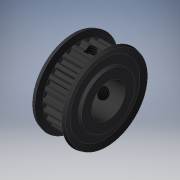
# Autodesk Inventor part: HTPA23S3M060-A-P10_b
Saved by Autodesk Inventor 2019 (Build 230136000, 136)
## iProperties
Created: 2022-11-04
Part Number: HTPA23S3M060-A-P10_b
Material: Generic
Catalog Web Link: www.cadenas.de
Description: HTPA__S3M060, HTPA__S3M100, HTPA__S3M150, HTPB__S3M060, HTPB__S3M100, HTPB__S3M150, HTPK__S3M060, HTPK__S3M100, HTPK__S3M150, HTPN__S3M060, HTPN__S3M100, HTPN__S3M150, HTPT__S3M060, HTPT__S3M100, HTPT__S3M150, HTPM__S3M060, HTPM__S3M100, HTPM__S3M150, HTPP__S3M060, HTPP__S3M100, HTPP__S3M150, HTPS__S3M060, HTPS__S3M100, KHTPA__S3M060, KHTPA__S3M100, KHTPA__S3M150, KHTPK__S3M060, KHTPK__S3M100, KHTPK__S3M150_body-High Torque Timing Pulleys S3M Type
Vendor: MISUMI
Document SubType Name: Modeling
Designer: psAdmin
Manufacturer: MISUMI
Mass: 2.63016 g
Surface Area: 24.7129 cm^2
Volume: 2.63016 cm^3
Density: 1 g/cm^3
Appearance: PSOLRGB-175-175-175
Category: PARTsolutions
Company: MISUMI
Title: HTPA23S3M060-A-P10
Author: Cadenas PARTsolutions
Comments: High Torque Timing Pulleys S3M Type
PSOL_IDENT_0: {$CADENAS_DATA/23d-libs/misumi/metric/51_timing_pulleys/htpk_s3m/htpa_s3m.prj},837 {VTYP=3D},{NB=HTP
PSOL_IDENT_1: A23S3M060-A-P10_b},{LINA=HTPA23S3M060-A-P10},{NN=HTPA__S3M060, HTPA__S3M100, HTPA__S3M150, HTPB__S3M
PSOL_IDENT_2: 060, HTPB__S3M100, HTPB__S3M150, HTPK__S3M060, HTPK__S3M100, HTPK__S3M150, HTPN__S3M060, HTPN__S3M10
PSOL_IDENT_3: 0, HTPN__S3M150, HTPT__S3M060, HTPT__S3M100, HTPT__S3M150, HTPM__S3M060, HTPM__S3M100, HTPM__S3M150,
PSOL_IDENT_4: HTPP__S3M060, HTPP__S3M100, HTPP__S3M150, HTPS__S3M060, HTPS__S3M100, KHTPA__S3M060, KHTPA__S3M100,
PSOL_IDENT_5: KHTPA__S3M150, KHTPK__S3M060, KHTPK__S3M100, KHTPK__S3M150_body},{DATE=28.10.2022 00:10:57},{GEOMDA
PSOL_IDENT_6: TE=11.11.2021 09:52:43},{VERSION=},{LINEID=330},{WBVAR=MATP,ST,TNW,PS,SBS,DD,Z,J,Q,R,S,T,ALT1,ALT2,M
PSOL_IDENT_7: ,QSC,QFC,QTC,ALT3,K,KSC,KFC,KTC,ALT4,ZM,ZSC,ZFC,ZTC,ALT5,ALT6,ALT7,FC,ALT8,SRG,ALT9,BTC,TL,ALT10,TPC
PSOL_IDENT_8: ,ALT11,BC,ALT12,SLH,ALT13,BN},{WBNUMERIC=DD,Z,J,Q,R,S,T,QSC,QFC,QTC,K,KSC,KFC,KTC,ZSC,ZFC,ZTC,FC,SRG
PSOL_IDENT_9: ,BTC,TL,BC,SLH,BN}  {NB=HTPA23S3M060-A-P10_b},{LINA=HTPA23S3M060-A-P10},{KT=DUMMY},{PN=HTPA23S3M060-
PSOL_IDENT_10: A-P10},{TYPE=HTPA},{MATP=A2017},{MATPALG='A2017','Aluminum Alloy 2000 series','S45C','1045 Carbon St
PSOL_IDENT_11: eel Equivalent','SUS304','304 Stainless Steel','A6000','6000 Series Aluminum Alloy'},{ST=CA},{STALG=
PSOL_IDENT_12: 'CA','Clear Anodize','BA','Black Anodize','HAT','Hard Clear Anodize','ENP','Electroless Nickel Plat
PSOL_IDENT_13: ing' },{NT=23},{TNW=S3M060},{TNWALG= 'S3M060','S3M100','S3M150'    },{BW=6},{PS=A},{PSALG='A','B'},{
PSOL_IDENT_14: SBS=P},{SBSALG= 'H','Round Hole','P','Round Hole + Tap','V','Stepped Hole', 'Y','Both Ends Stepped H
PSOL_IDENT_15: ole','WB', 'Double Stepped Hole' },{SHSA= 'H','Round Hole','P','Round Hole + Tap','V','Stepped Hole'
PSOL_IDENT_16: , 'Y','Both Ends Stepped Hole','WB', 'Double Stepped Hole' },{SHSB= 'H','Round Hole','P','Round Hole
PSOL_IDENT_17: + Tap','V','Stepped Hole','F','Stepped Hole (Counterbore holes on the boss side)'},{SHSK='H','Round
PSOL_IDENT_18: Hole','P','Round Hole + Tap'},{SBSPN=-P10},{DD=10.00},{DDALG=[4:4/1],4.5,[5:6/1],6.35,[7:10/1]},{DD
PSOL_IDENT_19: HA=[4:4/1],4.5,[5:6/1],6.35,[7:12/1]},{DDHBK=0},{DDPA=[4:4/1],4.5,[5:6/1],6.35,[7:10/1]},{DDPBK=0},{
PSOL_IDENT_20: DDNA=[8:8/1],[10:11/1]},{DDNBK=0},{DDNK=0},{DDCA=[10:10/1]},{DDCBK=0},{DDVA=[4:4/1],4.5,[5:6/1],6.35
PSOL_IDENT_21: ,[7:10/1]},{DDVF=[4:4/1],4.5,[5:6/1],6.35,[7:8/1]},{DDY=[4:10/1]},{DDWB=[4:8/1]},{Z=0},{ZALG=[0]},{Z
PSOL_IDENT_22: QRMIN=12},{ZAMAX=12},{ZBMAX=10},{DDZ=10},{J=0.0},{JALG=[0]},{JMAX=9},{JMIN=2},{JPN=},{QRMAX=12},{QRM
PSOL_IDENT_23: IN=12},{WBRMAX=-2.00},{WBQMIN=14},{Q=0},{QALG=[0]},{QPN=},{R=0},{RALG=[0]},{S=0.0},{SALG=[0]},{SPN=}
PSOL_IDENT_24: ,{SMAX=5},{T=0.0},{TALG=[0]},{TPN=},{TMAX=8},{A=7},{W=11},{L=0},{PD=21.96},{OD=21.20},{D=0},{DALG=25
PSOL_IDENT_25: },{DE=16},{F=25},{E=16},{BBK=0.000},{TTK=0.0},{TT=1},{ANG=125.217391},{WL=11},{ALT1=},{ALT1ALG= '','
PSOL_IDENT_26: w/o KC90 (Set Screw Angle)','KC90','with KC90 (Set Screw Angle)' },{ALT1PN=},{ALT2=},{ALT2ALG= '','N
PSOL_IDENT_27: ot applicable' },{M=N/A},{MALG= 'N/A' },{MFTALG= 'N/A' },{MSALG= 'N/A' },{M3D=0.000},{KDML=0},{ML=0}
PSOL_IDENT_28: ,{MUL=0},{PITCH=0},{QSC=0.0},{QSCALG=0},{QFC=0.0},{QFCALG=0},{QTC=0.0},{QTCALG=0},{QPCDMIN=0},{QPCDM
PSOL_IDENT_29: INALG=0},{QPCDMAX=12},{ALT2PN=},{ALT3=},{ALT3ALG= '','Not applicable' },{K=0.0},{KALG=0},{KMIN=4},{K
PSOL_IDENT_30: FTMAX=0.0},{KSMAX=0.0},{KSC=0.0},{KSCALG=0},{KFC=0.0},{KFCALG=0},{KTC=0.0},{KTCALG=0},{KPCDMIN=14},{
PSOL_IDENT_31: KPCDMINALG=14},{KPCDMAX=12},{KSCMIN=14.0},{KSCMINALG=14},{ALT3PN=},{ALT4=},{ALT4ALG= '','Not applica
PSOL_IDENT_32: ble' },{ALT4MIN=20.5},{ALT4MAX=5.5},{ZM=N/A},{ZMALG= 'N/A' },{ZMSALG= 'N/A' },{ZMFTALG= 'N/A' },{ZMD
PSOL_IDENT_33: D1=0.0},{ZMDD2=0.0},{ZMHH=0.0},{ZSC=0.0},{ZSCALG=[0]},{ZFC=0.0},{ZFCALG=[0]},{ZTC=0.0},{ZTCALG=[0]},
PSOL_IDENT_34: {ZPCDMIN=0},{ZPCDMINALG=0},{ZPCDMAX=12},{ALT4PN=},{ALT5=},{ALT5ALG= '','Flange Attached','NFC','with
PSOL_IDENT_35: NFC (Flange not Attached)' },{ALT5PN=},{ALT6=},{ALT6ALG= '','w/o Flange Attached on One Side Only','
PSOL_IDENT_36: RFC','with RFC (Flange Attached on The Boss Side Only)','LFC','with LFC (Flange Attached on The Oppo
PSOL_IDENT_37: site Side Only)' },{ALT6PN=},{ALT7=},{ALT7ALG= '','w/o FC (Flange Cut)','FC','with FC (Flange Cut)'
PSOL_IDENT_38: },{FC=0.0},{FCALG=0},{FCMIN=22.5},{FCMAX=23.0},{ALT7PN=},{ALT8=},{ALT8ALG= '','Not applicable' },{AL
PSOL_IDENT_39: T8ALGALG=12},{ALT8DD2=0},{ALT8MM=0},{ALT8NN=0},{QC=0},{KC=0},{ZC=0},{SRG=0.0},{SRGALG=[0]},{SRGMAX1=
PSOL_IDENT_40: 0},{SRGMAX=0},{DD2=0.0},{MM=0.00},{NN=0.00},{ALT8PN=},{ALT9ALG= '','w/o BTC (Taper for Bearing Holde
PSOL_IDENT_41: r)','BTC','with BTC (Taper for Bearing Holder)' },{ALT9=},{BTC9=11},{TL9=1},{BTC=0},{BTCALG=[0]},{TL=
PSOL_IDENT_42: 0.0},{TLALG=0},{TLMIN=1.0},{TLMAX=-11.5},{BTCL=0},{BTCD=0},{BTCDALG=16.000},{ALT9PN=},{WLBCTL=11},{A
PSOL_IDENT_43: LT10=},{ALT10ALG= '','w/o TPC (Tapped Hole Dimension)','TPC','with TPC (Tapped Hole Dimension)' },{T
PSOL_IDENT_44: PC=N/A},{TPCALG= 'N/A' },{TPCM=4},{ALT10PN=},{ALT11=},{ALT11ALG= '','Not applicable' },{BC=0.0},{BCA
PSOL_IDENT_45: LG=0},{BCMIN=7},{BCMAX=-11.5},{BCPLANE=5.5},{M1WBC=5.5},{ALT11PN=},{ALT12=},{ALT12ALG= '','w/o SLH (
PSOL_IDENT_46: Set Screw Length)','SLH','with SLH (Set Screw Length)' },{SLH=0},{SLHALG=[0]},{ALT12PN=},{AC=M4x3},{
PSOL_IDENT_47: M1=4},{M1L=3},{TAP=0.000},{KYY=5},{KTT=5.6},{PLANE=11},{CD=0},{ALT13=},{ALT13ALG= '', 'Not applicabl
PSOL_IDENT_48: e' },{BN=0.0},{BNALG=0},{BNMIN=-10.5},{BNMAX=-1.0},{ALT13PN=}
NB: HTPA23S3M060-A-P10_b
NN: 0
NT: 23
NBSYN: $PN._b
LINA: HTPA23S3M060-A-P10
CATALOG: Misumi
PN: HTPA23S3M060-A-P10
MATP: Aluminum Alloy 2000 series
ST: Clear Anodize
TNW: S3M060
BW: 6
PS: A
SBS: Round Hole + Tap
DD: 10
Z: 0
J: 0
Q: 0
R: 0
S: 0
T: 0
A: 7
W: 11
L: 0
PD: 21.96
OD: 21.2
D: 0
F: 25
E: 16
TT: 1
ALT1: w/o KC90 (Set Screw Angle)
ALT2: Not applicable
M: N/A
QSC: 0
QFC: 0
QTC: 0
ALT3: Not applicable
K: 0
KSC: 0
KFC: 0
KTC: 0
ALT4: Not applicable
ZM: N/A
ZMDD1: 0
ZMDD2: 0
ZMHH: 0
ZSC: 0
ZFC: 0
ZTC: 0
ALT5: Flange Attached
ALT6: w/o Flange Attached on One Side Only
ALT7: w/o FC (Flange Cut)
FC: 0
ALT8: Not applicable
SRG: 0
DD2: 0
MM: 0
ALT9: w/o BTC (Taper for Bearing Holder)
BTC: 0
TL: 0
BTCL: 0
BTCD: 0
ALT10: w/o TPC (Tapped Hole Dimension)
TPC: N/A
ALT11: Not applicable
BC: 0
ALT12: w/o SLH (Set Screw Length)
SLH: 0
AC: M4x3
ALT13: Not applicable
BN: 0
SUPPLIER: MISUMI
ARTICLENO: HTPA23S3M060-A-P10_b
BOMINFO: HTPA23S3M060-A-P10
CREATOR: CADENAS GmbH
Autodesk Inventor part; units mm, degrees
ref_plane "YZ Plane" through (0, 0, 0) normal (1, 0, 0) x (0, 1, 0)
ref_plane "XZ Plane" through (0, 0, 0) normal (0, 1, 0) x (-1, 0, 0)
ref_plane "XY Plane" through (0, 0, 0) normal (0, 0, 1) x (1, 0, 0)
sketch "_____1" plane through (0, 0, 0) normal (0, 0, 1) x (1, 0, 0)
  line L0 (11, 0) -> (0, 0)
  line L1 (0, 0) -> (0, 8)
  line L2 (0, 8) -> (1, 8)
  line L3 (1, 8) -> (1, 10.4683)
  line L4 (1, 10.4683) -> (0.525, 12.2412)
  line L5 (0.525, 12.2412) -> (1.4909, 12.5)
  line L6 (1.4909, 12.5) -> (2, 10.6)
  line L7 (2, 10.6) -> (9, 10.6)
  line L8 (9, 10.6) -> (9.5091, 12.5)
  line L9 (9.5091, 12.5) -> (10.475, 12.2412)
  line L10 (10.475, 12.2412) -> (10, 10.4683)
  line L11 (10, 10.4683) -> (10, 8)
  line L12 (10, 8) -> (11, 8)
  line L13 (11, 8) -> (11, 0)
  line L14 (11, 0) -> (0, 0)
  constraints: 30 end point
revolve "Revolution1" add sketch "_____1" angle 360 about axis through (11, 0, 0) along (1, 0, 0)
sketch "Sketch2" plane through (11, 0, 0) normal (1, 0, 0) x (0, 0, -1)
  point P0 (0, 0)
hole "Hole1" at (11, 0, 0) direction (-1, 0, 0) diameter 10 depth 11
sketch "_____6" plane through (2, 0, 0) normal (1, 0, 0) x (0, 0, -1)
  circle A0 centre (0, 0) radius 15.6
  arc A1 (-10.5889, 0.4842) -> (-10.3757, 0.1995) centre (-10.3092, 0.4715) ccw
  arc A2 (-9.534, -0.2416) -> (-10.3757, 0.1995) centre (-10.8446, -1.7191) ccw
  arc A3 (-9.4836, -0.3483) -> (-9.534, -0.2416) centre (-9.6335, -0.3538) ccw
  arc A4 (-9.4836, -0.3483) -> (-9.4427, -0.9463) centre (0, 0) ccw
  arc A5 (-9.4781, -1.0588) -> (-9.4427, -0.9463) centre (-9.592, -0.9612) ccw
  arc A6 (-10.2519, -1.6104) -> (-9.4781, -1.0588) centre (-10.9777, 0.2264) ccw
  arc A7 (-10.2519, -1.6104) -> (-10.4244, -1.9216) centre (-10.149, -1.8708) ccw
  arc A8 (-10.4244, -1.9216) -> (-10.3269, -2.3906) centre (0, 0) ccw
  arc A9 (-10.3269, -2.3906) -> (-10.0448, -2.6073) centre (-10.0541, -2.3274) ccw
  arc A10 (-9.1152, -2.8049) -> (-10.0448, -2.6073) centre (-9.9786, -4.5812) ccw
  arc A11 (-9.038, -2.894) -> (-9.1152, -2.8049) centre (-9.1808, -2.9398) ccw
  arc A12 (-9.038, -2.894) -> (-8.8372, -3.4588) centre (0, 0) ccw
  arc A13 (-8.8409, -3.5767) -> (-8.8372, -3.4588) centre (-8.9769, -3.5135) ccw
  arc A14 (-9.4372, -4.3166) -> (-8.8409, -3.5767) centre (-10.6317, -2.7437) ccw
  arc A15 (-9.4372, -4.3166) -> (-9.5194, -4.6628) centre (-9.2679, -4.5396) ccw
  arc A16 (-9.5194, -4.6628) -> (-9.299, -5.0881) centre (0, 0) ccw
  arc A17 (-9.299, -5.0881) -> (-8.9688, -5.2206) centre (-9.0534, -4.9537) ccw
  arc A18 (-8.0205, -5.1601) -> (-8.9688, -5.2206) centre (-8.3726, -7.1035) ccw
  arc A19 (-7.922, -5.2251) -> (-8.0205, -5.1601) centre (-8.0472, -5.3077) ccw
  arc A20 (-7.922, -5.2251) -> (-7.5764, -5.7148) centre (0, 0) ccw
  arc A21 (-7.5481, -5.8293) -> (-7.5764, -5.7148) centre (-7.6961, -5.8051) ccw
  arc A22 (-7.9227, -6.7027) -> (-7.5481, -5.8293) centre (-9.4972, -5.5104) ccw
  arc A23 (-7.9227, -6.7027) -> (-7.9084, -7.0582) centre (-7.6995, -6.8717) ccw
  arc A24 (-7.9084, -7.0582) -> (-7.5814, -7.4082) centre (0, 0) ccw
  arc A25 (-7.5814, -7.4082) -> (-7.2277, -7.4468) centre (-7.3812, -7.2126) ccw
  arc A26 (-6.3309, -7.1327) -> (-7.2277, -7.4468) centre (-6.1457, -9.099) ccw
  arc A27 (-6.2185, -7.1687) -> (-6.3309, -7.1327) centre (-6.3168, -7.282) ccw
  arc A28 (-6.2185, -7.1687) -> (-5.7536, -7.547) centre (0, 0) ccw
  arc A29 (-5.6954, -7.6496) -> (-5.7536, -7.547) centre (-5.8445, -7.6662) ccw
  arc A30 (-5.8205, -8.5917) -> (-5.6954, -7.6496) centre (-7.6583, -7.8684) ccw
  arc A31 (-5.8205, -8.5917) -> (-5.7108, -8.9301) centre (-5.56, -8.6942) ccw
  arc A32 (-5.7108, -8.9301) -> (-5.3016, -9.179) centre (0, 0) ccw
  arc A33 (-5.3016, -9.179) -> (-4.9506, -9.1207) centre (-5.1615, -8.9365) ccw
  arc A34 (-4.1717, -8.5762) -> (-4.9506, -9.1207) centre (-3.4629, -10.4196) ccw
  arc A35 (-4.0538, -8.5806) -> (-4.1717, -8.5762) centre (-4.1179, -8.7162) ccw
  arc A36 (-4.0538, -8.5806) -> (-3.5041, -8.8194) centre (0, 0) ccw
  arc A37 (-3.4204, -8.9026) -> (-3.5041, -8.8194) centre (-3.5595, -8.9588) ccw
  arc A38 (-3.2867, -9.8434) -> (-3.4204, -8.9026) centre (-5.2514, -9.6428) ccw
  arc A39 (-3.2867, -9.8434) -> (-3.0897, -10.1397) centre (-3.0081, -9.8719) ccw
  arc A40 (-3.0897, -10.1397) -> (-2.6285, -10.2689) centre (0, 0) ccw
  arc A41 (-2.6285, -10.2689) -> (-2.3063, -10.1181) centre (-2.5591, -9.9977) ccw
  arc A42 (-1.7032, -9.3837) -> (-2.3063, -10.1181) centre (-0.5233, -10.9675) ccw
  arc A43 (-1.5885, -9.3561) -> (-1.7032, -9.3837) centre (-1.6136, -9.504) ccw
  arc A44 (-1.5885, -9.3561) -> (-0.9947, -9.4377) centre (0, 0) ccw
  arc A45 (-0.8917, -9.4952) -> (-0.9947, -9.4377) centre (-1.0104, -9.5869) ccw
  arc A46 (-0.5091, -10.3651) -> (-0.8917, -9.4952) centre (-2.4551, -10.702) ccw
  arc A47 (-0.5091, -10.3651) -> (-0.2395, -10.5973) centre (-0.2332, -10.3174) ccw
  arc A48 (-0.2395, -10.5973) -> (0.2395, -10.5973) centre (0, 0) ccw
  arc A49 (0.2395, -10.5973) -> (0.5091, -10.3651) centre (0.2332, -10.3174) ccw
  arc A50 (0.8917, -9.4952) -> (0.5091, -10.3651) centre (2.4551, -10.702) ccw
  arc A51 (0.9947, -9.4377) -> (0.8917, -9.4952) centre (1.0104, -9.5869) ccw
  arc A52 (0.9947, -9.4377) -> (1.5885, -9.3561) centre (0, 0) ccw
  arc A53 (1.7032, -9.3837) -> (1.5885, -9.3561) centre (1.6136, -9.504) ccw
  arc A54 (2.3063, -10.1181) -> (1.7032, -9.3837) centre (0.5233, -10.9675) ccw
  arc A55 (2.3063, -10.1181) -> (2.6285, -10.2689) centre (2.5591, -9.9977) ccw
  arc A56 (2.6285, -10.2689) -> (3.0897, -10.1397) centre (0, 0) ccw
  arc A57 (3.0897, -10.1397) -> (3.2867, -9.8434) centre (3.0081, -9.8719) ccw
  arc A58 (3.4204, -8.9026) -> (3.2867, -9.8434) centre (5.2514, -9.6428) ccw
  arc A59 (3.5041, -8.8194) -> (3.4204, -8.9026) centre (3.5595, -8.9588) ccw
  arc A60 (3.5041, -8.8194) -> (4.0538, -8.5806) centre (0, 0) ccw
  arc A61 (4.1717, -8.5762) -> (4.0538, -8.5806) centre (4.1179, -8.7162) ccw
  arc A62 (4.9506, -9.1207) -> (4.1717, -8.5762) centre (3.4629, -10.4196) ccw
  arc A63 (4.9506, -9.1207) -> (5.3016, -9.179) centre (5.1615, -8.9365) ccw
  arc A64 (5.3016, -9.179) -> (5.7108, -8.9301) centre (0, 0) ccw
  arc A65 (5.7108, -8.9301) -> (5.8205, -8.5917) centre (5.56, -8.6942) ccw
  arc A66 (5.6954, -7.6496) -> (5.8205, -8.5917) centre (7.6583, -7.8684) ccw
  arc A67 (5.7536, -7.547) -> (5.6954, -7.6496) centre (5.8445, -7.6662) ccw
  arc A68 (5.7536, -7.547) -> (6.2185, -7.1687) centre (0, 0) ccw
  arc A69 (6.3309, -7.1327) -> (6.2185, -7.1687) centre (6.3168, -7.282) ccw
  arc A70 (7.2277, -7.4468) -> (6.3309, -7.1327) centre (6.1457, -9.099) ccw
  arc A71 (7.2277, -7.4468) -> (7.5814, -7.4082) centre (7.3812, -7.2126) ccw
  arc A72 (7.5814, -7.4082) -> (7.9084, -7.0582) centre (0, 0) ccw
  arc A73 (7.9084, -7.0582) -> (7.9227, -6.7027) centre (7.6995, -6.8717) ccw
  arc A74 (7.5481, -5.8293) -> (7.9227, -6.7027) centre (9.4972, -5.5104) ccw
  arc A75 (7.5764, -5.7148) -> (7.5481, -5.8293) centre (7.6961, -5.8051) ccw
  arc A76 (7.5764, -5.7148) -> (7.922, -5.2251) centre (0, 0) ccw
  arc A77 (8.0205, -5.1601) -> (7.922, -5.2251) centre (8.0472, -5.3077) ccw
  arc A78 (8.9688, -5.2206) -> (8.0205, -5.1601) centre (8.3726, -7.1035) ccw
  arc A79 (8.9688, -5.2206) -> (9.299, -5.0881) centre (9.0534, -4.9537) ccw
  arc A80 (9.299, -5.0881) -> (9.5194, -4.6628) centre (0, 0) ccw
  arc A81 (9.5194, -4.6628) -> (9.4372, -4.3166) centre (9.2679, -4.5396) ccw
  arc A82 (8.8409, -3.5767) -> (9.4372, -4.3166) centre (10.6317, -2.7437) ccw
  arc A83 (8.8372, -3.4588) -> (8.8409, -3.5767) centre (8.9769, -3.5135) ccw
  arc A84 (8.8372, -3.4588) -> (9.038, -2.894) centre (0, 0) ccw
  arc A85 (9.1152, -2.8049) -> (9.038, -2.894) centre (9.1808, -2.9398) ccw
  arc A86 (10.0448, -2.6073) -> (9.1152, -2.8049) centre (9.9786, -4.5812) ccw
  arc A87 (10.0448, -2.6073) -> (10.3269, -2.3906) centre (10.0541, -2.3274) ccw
  arc A88 (10.3269, -2.3906) -> (10.4244, -1.9216) centre (0, 0) ccw
  arc A89 (10.4244, -1.9216) -> (10.2519, -1.6104) centre (10.149, -1.8708) ccw
  arc A90 (9.4781, -1.0588) -> (10.2519, -1.6104) centre (10.9777, 0.2264) ccw
  arc A91 (9.4427, -0.9463) -> (9.4781, -1.0588) centre (9.592, -0.9612) ccw
  arc A92 (9.4427, -0.9463) -> (9.4836, -0.3483) centre (0, 0) ccw
  arc A93 (9.534, -0.2416) -> (9.4836, -0.3483) centre (9.6335, -0.3538) ccw
  arc A94 (10.3757, 0.1995) -> (9.534, -0.2416) centre (10.8446, -1.7191) ccw
  arc A95 (10.3757, 0.1995) -> (10.5889, 0.4842) centre (10.3092, 0.4715) ccw
  arc A96 (10.5889, 0.4842) -> (10.5562, 0.9621) centre (0, 0) ccw
  arc A97 (10.5562, 0.9621) -> (10.3062, 1.2152) centre (10.2774, 0.9367) ccw
  arc A98 (9.4123, 1.5376) -> (10.3062, 1.2152) centre (10.5095, 3.1797) ccw
  arc A99 (9.3478, 1.6364) -> (9.4123, 1.5376) centre (9.4956, 1.6623) ccw
  arc A100 (9.3478, 1.6364) -> (9.2259, 2.2232) centre (0, 0) ccw
  arc A101 (9.2456, 2.3396) -> (9.2259, 2.2232) centre (9.3717, 2.2584) ccw
  arc A102 (9.9371, 2.9914) -> (9.2456, 2.3396) centre (10.9062, 1.2705) ccw
  arc A103 (9.9371, 2.9914) -> (10.0656, 3.3232) centre (9.7997, 3.2354) ccw
  arc A104 (10.0656, 3.3232) -> (9.9052, 3.7745) centre (0, 0) ccw
  arc A105 (9.9052, 3.7745) -> (9.5962, 3.9507) centre (9.6436, 3.6748) ccw
  arc A106 (8.6484, 4.02) -> (9.5962, 3.9507) centre (9.2619, 5.8972) ccw
  arc A107 (8.5597, 4.0978) -> (8.6484, 4.02) centre (8.695, 4.1625) ccw
  arc A108 (8.5597, 4.0978) -> (8.284, 4.6299) centre (0, 0) ccw
  arc A109 (8.2715, 4.7473) -> (8.284, 4.6299) centre (8.4149, 4.7031) ccw
  arc A110 (8.7616, 5.5615) -> (8.2715, 4.7473) centre (10.159, 4.1659) ccw
  arc A111 (8.7616, 5.5615) -> (8.7958, 5.9156) centre (8.5634, 5.7593) ccw
  arc A112 (8.7958, 5.9156) -> (8.5196, 6.3069) centre (0, 0) ccw
  arc A113 (8.5196, 6.3069) -> (8.1744, 6.3933) centre (8.2945, 6.1403) ccw
  arc A114 (7.2431, 6.2042) -> (8.1744, 6.3933) centre (7.3274, 8.1774) ccw
  arc A115 (7.1367, 6.2552) -> (7.2431, 6.2042) centre (7.2495, 6.3541) ccw
  arc A116 (7.1367, 6.2552) -> (6.7276, 6.6932) centre (0, 0) ccw
  arc A117 (6.684, 6.8028) -> (6.7276, 6.6932) centre (6.834, 6.799) ccw
  arc A118 (6.9362, 7.7191) -> (6.684, 6.8028) centre (8.6584, 6.7523) ccw
  arc A119 (6.9362, 7.7191) -> (6.8736, 8.0693) centre (6.692, 7.8561) ccw
  arc A120 (6.8736, 8.0693) -> (6.502, 8.3716) centre (0, 0) ccw
  arc A121 (6.502, 8.3716) -> (6.1464, 8.3616) centre (6.3303, 8.1504) ccw
  arc A122 (5.3007, 7.9283) -> (6.1464, 8.3616) centre (4.8494, 9.8511) ccw
  arc A123 (5.1844, 7.9487) -> (5.3007, 7.9283) centre (5.2664, 8.0743) ccw
  arc A124 (5.1844, 7.9487) -> (4.6723, 8.2601) centre (0, 0) ccw
  arc A125 (4.6008, 8.3539) -> (4.6723, 8.2601) centre (4.7462, 8.3907) ccw
  arc A126 (4.5964, 9.3042) -> (4.6008, 8.3539) centre (6.5156, 8.8379) ccw
  arc A127 (4.5964, 9.3042) -> (4.4416, 9.6245) centre (4.3243, 9.3703) ccw
  arc A128 (4.4416, 9.6245) -> (4.0023, 9.8154) centre (0, 0) ccw
  arc A129 (4.0023, 9.8154) -> (3.6626, 9.7098) centre (3.8966, 9.5561) ccw
  arc A130 (2.9651, 9.0644) -> (3.6626, 9.7098) centre (2.0118, 10.7941) ccw
  arc A131 (2.8477, 9.0527) -> (2.9651, 9.0644) centre (2.8927, 9.1958) ccw
  arc A132 (2.8477, 9.0527) -> (2.2705, 9.2144) centre (0, 0) ccw
  arc A133 (2.1763, 9.2854) -> (2.2705, 9.2144) centre (2.3064, 9.36) ccw
  arc A134 (1.9157, 10.1993) -> (2.1763, 9.2854) centre (3.8895, 10.268) ccw
  arc A135 (1.9157, 10.1993) -> (1.6803, 10.466) centre (1.6359, 10.1895) ccw
  arc A136 (1.6803, 10.466) -> (1.2057, 10.5312) centre (0, 0) ccw
  arc A137 (1.2057, 10.5312) -> (0.9071, 10.3379) centre (1.1739, 10.253) ccw
  arc A138 (0.4096, 9.5282) -> (0.9071, 10.3379) centre (-0.975, 10.9366) ccw
  arc A139 (0.2997, 9.4853) -> (0.4096, 9.5282) centre (0.3044, 9.6352) ccw
  arc A140 (0.2997, 9.4853) -> (-0.2997, 9.4853) centre (0, 0) ccw
  arc A141 (-0.4096, 9.5282) -> (-0.2997, 9.4853) centre (-0.3044, 9.6352) ccw
  arc A142 (-0.9071, 10.3379) -> (-0.4096, 9.5282) centre (0.975, 10.9366) ccw
  arc A143 (-0.9071, 10.3379) -> (-1.2057, 10.5312) centre (-1.1739, 10.253) ccw
  arc A144 (-1.2057, 10.5312) -> (-1.6803, 10.466) centre (0, 0) ccw
  arc A145 (-1.6803, 10.466) -> (-1.9157, 10.1993) centre (-1.6359, 10.1895) ccw
  arc A146 (-2.1763, 9.2854) -> (-1.9157, 10.1993) centre (-3.8895, 10.268) ccw
  arc A147 (-2.2705, 9.2144) -> (-2.1763, 9.2854) centre (-2.3064, 9.36) ccw
  arc A148 (-2.2705, 9.2144) -> (-2.8477, 9.0527) centre (0, 0) ccw
  arc A149 (-2.9651, 9.0644) -> (-2.8477, 9.0527) centre (-2.8927, 9.1958) ccw
  arc A150 (-3.6626, 9.7098) -> (-2.9651, 9.0644) centre (-2.0118, 10.7941) ccw
  arc A151 (-3.6626, 9.7098) -> (-4.0023, 9.8154) centre (-3.8966, 9.5561) ccw
  arc A152 (-4.0023, 9.8154) -> (-4.4416, 9.6245) centre (0, 0) ccw
  arc A153 (-4.4416, 9.6245) -> (-4.5964, 9.3042) centre (-4.3243, 9.3703) ccw
  arc A154 (-4.6008, 8.3539) -> (-4.5964, 9.3042) centre (-6.5156, 8.8379) ccw
  arc A155 (-4.6723, 8.2601) -> (-4.6008, 8.3539) centre (-4.7462, 8.3907) ccw
  arc A156 (-4.6723, 8.2601) -> (-5.1844, 7.9487) centre (0, 0) ccw
  arc A157 (-5.3007, 7.9283) -> (-5.1844, 7.9487) centre (-5.2664, 8.0743) ccw
  arc A158 (-6.1464, 8.3616) -> (-5.3007, 7.9283) centre (-4.8494, 9.8511) ccw
  arc A159 (-6.1464, 8.3616) -> (-6.502, 8.3716) centre (-6.3303, 8.1504) ccw
  arc A160 (-6.502, 8.3716) -> (-6.8736, 8.0693) centre (0, 0) ccw
  arc A161 (-6.8736, 8.0693) -> (-6.9362, 7.7191) centre (-6.692, 7.8561) ccw
  arc A162 (-6.684, 6.8028) -> (-6.9362, 7.7191) centre (-8.6584, 6.7523) ccw
  arc A163 (-6.7276, 6.6932) -> (-6.684, 6.8028) centre (-6.834, 6.799) ccw
  arc A164 (-6.7276, 6.6932) -> (-7.1367, 6.2552) centre (0, 0) ccw
  arc A165 (-7.2431, 6.2042) -> (-7.1367, 6.2552) centre (-7.2495, 6.3541) ccw
  arc A166 (-8.1744, 6.3933) -> (-7.2431, 6.2042) centre (-7.3274, 8.1774) ccw
  arc A167 (-8.1744, 6.3933) -> (-8.5196, 6.3069) centre (-8.2945, 6.1403) ccw
  arc A168 (-8.5196, 6.3069) -> (-8.7958, 5.9156) centre (0, 0) ccw
  arc A169 (-8.7958, 5.9156) -> (-8.7616, 5.5615) centre (-8.5634, 5.7593) ccw
  arc A170 (-8.2715, 4.7473) -> (-8.7616, 5.5615) centre (-10.159, 4.1659) ccw
  arc A171 (-8.284, 4.6299) -> (-8.2715, 4.7473) centre (-8.4149, 4.7031) ccw
  arc A172 (-8.284, 4.6299) -> (-8.5597, 4.0978) centre (0, 0) ccw
  arc A173 (-8.6484, 4.02) -> (-8.5597, 4.0978) centre (-8.695, 4.1625) ccw
  arc A174 (-9.5962, 3.9507) -> (-8.6484, 4.02) centre (-9.2619, 5.8972) ccw
  arc A175 (-9.5962, 3.9507) -> (-9.9052, 3.7745) centre (-9.6436, 3.6748) ccw
  arc A176 (-9.9052, 3.7745) -> (-10.0656, 3.3232) centre (0, 0) ccw
  arc A177 (-10.0656, 3.3232) -> (-9.9371, 2.9914) centre (-9.7997, 3.2354) ccw
  arc A178 (-9.2456, 2.3396) -> (-9.9371, 2.9914) centre (-10.9062, 1.2705) ccw
  arc A179 (-9.2259, 2.2232) -> (-9.2456, 2.3396) centre (-9.3717, 2.2584) ccw
  arc A180 (-9.2259, 2.2232) -> (-9.3478, 1.6364) centre (0, 0) ccw
  arc A181 (-9.4123, 1.5376) -> (-9.3478, 1.6364) centre (-9.4956, 1.6623) ccw
  arc A182 (-10.3062, 1.2152) -> (-9.4123, 1.5376) centre (-10.5095, 3.1797) ccw
  arc A183 (-10.3062, 1.2152) -> (-10.5562, 0.9621) centre (-10.2774, 0.9367) ccw
  arc A184 (-10.5562, 0.9621) -> (-10.5889, 0.4842) centre (0, 0) ccw
  constraints: 368 point on circle, 185 centre point
extrude "Extrusion1" cut sketch "_____6" along normal blind 7
sketch "_____18" plane through (5.5, 0, 0) normal (1, 0, 0) x (0, 0, -1)
  line L0 (0, 0) -> (0, 10.6)
  line L1 (0, 10.6) -> (1.621, 10.6)
  line L2 (1.621, 10.6) -> (1.621, 0)
  line L3 (1.621, 0) -> (0, 0)
  line L4 (0, 0) -> (0, 10.6)
  constraints: 10 end point
revolve "Revolution2" cut sketch "_____18" angle 360 about axis through (5.5, 0, 0) along (0, -1, 0)
thread "Thread1" size "M4x0.7" class "6H" standard "ISO Metric profile" length 5.6
sketch "_____19" plane through (5.5, 0, 0) normal (1, 0, 0) x (0, 0, -1)
  line L0 (0, 0) -> (8.6599, -6.1128)
  line L1 (8.6599, -6.1128) -> (7.7251, -7.4371)
  line L2 (7.7251, -7.4371) -> (-0.9348, -1.3243)
  line L3 (-0.9348, -1.3243) -> (0, 0)
  line L4 (0, 0) -> (8.6599, -6.1128)
  constraints: 10 end point
revolve "Revolution3" cut sketch "_____19" angle 360 about axis through (5.5, 0, 0) along (0, 0.5766803, 0.8169699)
thread "Thread2" size "M4x0.7" class "6H" standard "ISO Metric profile" length 5.6 offset 0.1454
ref_plane "to_belt_XY" through (5.5, 0, 0) normal (-1, 0, 0) x (0, 0, -1)
ref_plane "to_belt_YZ" through (5.5, 0, 0) normal (0, 0, -1) x (0, -1, 0)
ref_plane "to_belt_ZX" through (5.5, 0, 0) normal (0, -1, 0) x (-1, 0, 0)
ref_plane "to_screw1_XY" through (5.5, 5, 0) normal (0, 1, 0) x (1, 0, 0)
ref_plane "to_screw1_YZ" through (5.5, 5, 0) normal (1, 0, 0) x (0, 0, -1)
ref_plane "to_screw1_ZX" through (5.5, 5, 0) normal (0, 0, -1) x (0, 1, 0)
ref_plane "to_screw2_XY" through (5.5, -2.8834, -4.0848) normal (0, -0.5766803, -0.8169699) x (1, 0, 0)
ref_plane "to_screw2_YZ" through (5.5, -2.8834, -4.0848) normal (1, 0, 0) x (0, -0.8169699, 0.5766803)
ref_plane "to_screw2_ZX" through (5.5, -2.8834, -4.0848) normal (0, -0.8169699, 0.5766803) x (0, -0.5766803, -0.8169699)
body "Solid1"
